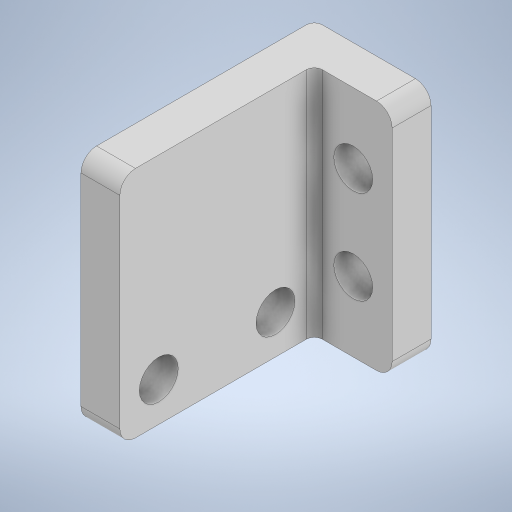
# Autodesk Inventor part: BP_BOX-Support-Bar-Connect1
Saved by Autodesk Inventor 2024.3 (Build 283343000, 343)
## iProperties
Created: 2025-11-18
Part Number: BP_BOX-Support-Bar-Connect1
Material: 一般
Document SubType Name: Modeling
Designer: 佐藤智貴
Density: 1 g/cm^3
Appearance: 既定
Author: 佐藤智貴
Autodesk Inventor part; units mm, degrees
ref_plane "YZ Plane" through (0, 0, 0) normal (1, 0, 0) x (0, 1, 0)
ref_plane "XZ Plane" through (0, 0, 0) normal (0, 1, 0) x (-1, 0, 0)
ref_plane "XY Plane" through (0, 0, 0) normal (0, 0, 1) x (1, 0, 0)
sketch "スケッチ1" plane through (0, 0, 0) normal (0, 0, 1) x (1, 0, 0)
  line L0 (0, 0) -> (5, 0)
  line L1 (5, 0) -> (5, 30)
  line L2 (5, 30) -> (0, 30)
  line L3 (0, 30) -> (0, 0)
  line L4 (5, 30) -> (15, 30)
  line L5 (15, 30) -> (15, 0)
  line L6 (15, 0) -> (5, 0)
  line L7 (5, 0) -> (5, 30)
  dimension "d0" = 30
  dimension "d1" = 5
  dimension "d2" = 30
  dimension "d3" = 10
  constraints: 16 end point, 4 parallel, 2 horizontal, 2 perpendicular
  measures "d0" distance of L0.end L1.end
  measures "d1" distance of L1.end L2.end
  measures "d2" distance of L4.end L5.end
  measures "d3" distance between parallel lines of L1 L5
extrude "押し出し1" add sketch "スケッチ1" along normal blind 5
sketch "スケッチ2" plane through (0, 0, 5) normal (0, 0, 1) x (1, 0, 0)
  line L0 (15, 0) -> (15, 30) projected
  line L1 (0, 0) -> (15, 0) projected
  line L2 (15, 30) -> (5, 30)
  line L3 (5, 30) -> (5, 0)
  line L4 (5, 0) -> (15, 0)
  line L5 (15, 0) -> (15, 30)
  point P0 (10, 21)
  point P1 (10, 9)
  dimension "d6" = 10
  dimension "d7" = 5
  dimension "d8" = 9
  dimension "d9" = 9
  dimension "d10" = 5
  constraints: 8 end point, 2 parallel, 1 horizontal, 1 perpendicular, 1 point on line
  measures "d6" distance between parallel lines of L0 L3
  measures "d7" distance from line of L5 point (10, 9)
  measures "d8" distance from line of L1 point (10, 9)
  measures "d9" distance from line of L2 point (10, 21)
  measures "d10" distance from line of L0 point (10, 21)
hole "穴1" at (10, 21, 5) at (10, 9, 5) direction (0, 0, -1) diameter 5 depth 8
sketch "スケッチ3" plane through (0, 0, 5) normal (0, 0, 1) x (1, 0, 0)
  line L0 (15, 30) -> (0, 30) projected
  line L1 (0, 0) -> (15, 0) projected
  line L2 (0, 30) -> (5, 30)
  line L3 (5, 30) -> (5, 0)
  line L4 (5, 0) -> (0, 0)
  line L5 (0, 0) -> (0, 30)
  dimension "d18" = 5
  constraints: 8 end point, 2 parallel, 1 horizontal, 1 perpendicular, 1 point on line
  measures "d18" distance between parallel lines of L5 L3
extrude "押し出し2" add sketch "スケッチ3" along normal blind 30
sketch "スケッチ4" plane through (5, 0, 5) normal (1, 0, 0) x (0, 0, -1)
  line L0 (-30, 0) -> (-30, 30) projected
  line L1 (0, 0) -> (-30, 0) projected
  line L2 (5, 0) -> (5, 30) projected
  point P0 (-20, 5)
  point P1 (-5, 5)
  dimension "d21" = 15
  dimension "d22" = 10
  dimension "d23" = 5
  dimension "d24" = 5
  dimension "d25" = 10
  measures "d21" distance of point (-20, 5) point (-5, 5)
  measures "d22" distance from line of L0 point (-20, 5)
  measures "d23" distance from line of L1 point (-20, 5)
  measures "d24" distance from line of L1 point (-5, 5)
  measures "d25" distance from line of L2 point (-5, 5)
hole "穴2" at (5, 5, 25) at (5, 5, 10) direction (-1, 0, 0) diameter 5 depth 8
sketch "スケッチ5" plane through (5, 0, 5) normal (1, 0, 0) x (0, 0, -1)
  line L0 (5, 30) -> (-30, 30) projected
  line L1 (-30, 30) -> (-25, 30)
  line L2 (-25, 30) -> (-25, 0)
  line L3 (-25, 0) -> (-30, 0)
  line L4 (-30, 0) -> (-30, 30)
  line L5 (0, 0) -> (0, 30) projected
  circle A0 centre (-5, 5) radius 2.5 projected
  circle A1 centre (-20, 5) radius 2.5 projected
  point P0 (5, 0)
  dimension "d33" = 5
  dimension "d34" = 5
  constraints: 8 end point, 2 parallel, 1 horizontal, 1 perpendicular
  measures "d33" distance from line of L5 A0.centre
  measures "d34" distance from line of A1.centre L2
extrude "押し出し3" cut sketch "スケッチ5" against normal through all contours L2 L3 L4 L0
fillet "フィレット1" radius 2 4 edges at (2.5, 30, 30) (2.5, 0, 30) (15, 30, 2.5) (15, 0, 2.5)
fillet "フィレット2" radius 1 2 edges at (0, 15, 0) (5, 15, 5)
equation "\"d9\" = d8"
equation "\"d10\" = d7"
equation "\"d24\" = d23"
equation "\"d34\" = d33"
